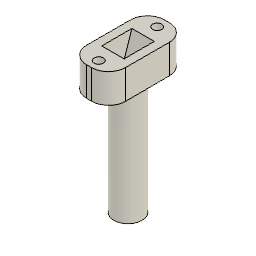
Shroud 3mm (Autodesk Fusion 360 design; units mm, degrees)
Autodesk Fusion 360 part; units mm, degrees
sketch "Sketch1" plane through (0, 0, 0) normal (0, 0, 1) x (1, 0, 0)
  circle A0 centre (0, 0) radius 1.9
  circle A1 centre (0, 0) radius 2.9
  dimension "d1" = 3.8
  dimension "d2" = 5.8
  constraint coincident A0.centre A1.centre
  measures "d1" diameter of A0
  measures "d2" diameter of A1
extrude "Extrude1" add sketch "Sketch1" along normal blind 7
sketch "Sketch2" plane through (0, 0, 7) normal (0, 0, 1) x (-1, 0, 0)
  circle A0 centre (0, 0) radius 1.9
  circle A1 centre (0, 0) radius 2.9
  line L0 (-2.3, 1.1) -> (2.3, 1.1)
  line L1 (2.3, 1.1) -> (2.3, -1.1)
  line L2 (2.3, -1.1) -> (-2.3, -1.1)
  line L3 (-2.3, -1.1) -> (-2.3, 1.1)
  line L4 (-2.3, 1.1) -> (2.3, -1.1) construction
  line L5 (2.3, 1.1) -> (-2.3, -1.1) construction
  line L6 (-4, 8) -> (4, 8)
  line L7 (4, 8) -> (4, -8)
  line L8 (4, -8) -> (-4, -8)
  line L9 (-4, -8) -> (-4, 8)
  line L10 (-4, 8) -> (4, -8) construction
  line L11 (4, 8) -> (-4, -8) construction
  dimension "d5" = 4.6
  dimension "d6" = 2.2
  dimension "d7" = 8
  dimension "d8" = 16
  constraint horizontal L0
  constraint perpendicular L0 L1
  constraint parallel L0 L2
  constraint parallel L1 L3
  constraint coincident L4 A0.centre
  constraint coincident L5 A0.centre
  constraint coincident A0.centre A1.centre
  constraint horizontal L6
  constraint perpendicular L6 L7
  constraint parallel L6 L8
  constraint parallel L7 L9
  constraint coincident L10 A0.centre
  constraint coincident L11 A0.centre
  measures "d5" distance of L1.end L2.end
  measures "d6" distance of L0.end L1.end
  measures "d7" distance of L7.end L8.end
  measures "d8" distance of L6.end L7.end
extrude "Extrude2" add sketch "Sketch2" along normal blind 23 contours A0 L0 | A0 L2 | A1 | L6 L7 L8 L9
sketch "Sketch3" plane through (0, 0, 30) normal (0, 0, 1) x (-1, 0, 0)
  line L0 (2.3, -1.1) -> (-2.3, -1.1)
  line L1 (-2.3, -1.1) -> (-2.3, 1.1)
  line L2 (-2.3, 1.1) -> (2.3, 1.1)
  line L3 (2.3, 1.1) -> (2.3, -1.1)
  line L4 (-4, -8) -> (4, -8)
  line L5 (4, -8) -> (4, 8)
  line L6 (4, 8) -> (-4, 8)
  line L7 (-4, 8) -> (-4, -8)
  circle A0 centre (0, -6) radius 0.95
  circle A1 centre (0, 6) radius 0.95
  line L8 (5, 0) -> (-5, 0) construction
  line L9 (0, -10) -> (0, 10) construction
  dimension "d11" = 1.9
  dimension "d12" = 1.9
  dimension "d13" = 6
  dimension "d14" = 6
  constraint perpendicular L3 L8
  constraint perpendicular L6 L9
  measures "d11" diameter of A0
  measures "d12" diameter of A1
  measures "d13" distance of A0.centre L8
  measures "d14" distance of A1.centre L8
fillet "Fillet1" radius 3.5 4 edges at (4, 8, 18.5) (4, -8, 18.5) (-4, -8, 18.5) (-4, 8, 18.5)
extrude "Extrude3" cut sketch "Sketch3" against normal blind 23 contours A0 | A1
move_face "OffsetFaces1" offset -17 1 faces at (2.0488, -4.1218, 7)
chamfer "Chamfer1" distance 0.5 angle 45 1 edges at (-1.7714, 0.6871, 0)
fillet "Fillet2" radius 1 2 edges at (-2.7037, -1.0487, 24) (-2.7037, -1.0487, 24)
chamfer "Chamfer2" distance 2 distance2 6 2 edges at (0, 1.1, 30) (0, -1.1, 30) measured on face at (0.0237, 2.4176, 30) measured on face at (0.0237, 2.4176, 30)
